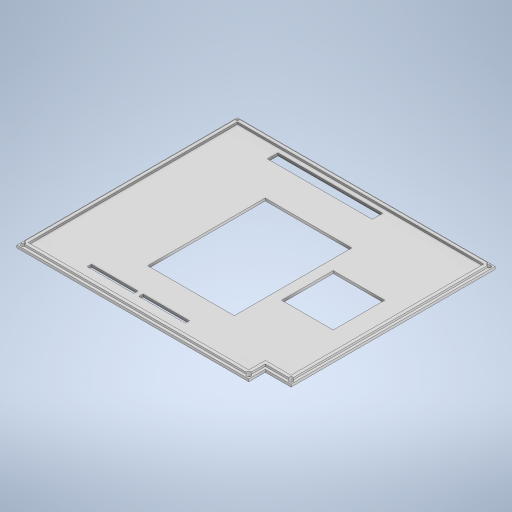
# Autodesk Inventor part: Xavier V3-1 Lid
Saved by Autodesk Inventor 2024 (Build 280153000, 153)
## iProperties
Created: 2023-11-29
Part Number: Xavier V3-1 Lid
Material: Generic
Document SubType Name: Modeling
Designer: close
Density: 1 g/cm^3
Appearance: Default
Author: close
Autodesk Inventor part; units mm, degrees
ref_plane "YZ Plane" through (0, 0, 0) normal (1, 0, 0) x (0, 1, 0)
ref_plane "XZ Plane" through (0, 0, 0) normal (0, 1, 0) x (-1, 0, 0)
ref_plane "XY Plane" through (0, 0, 0) normal (0, 0, 1) x (1, 0, 0)
sketch "Sketch1" plane through (0, 0, 0) normal (0, 1, 0) x (-1, 0, 0)
  line L0 (0, 0) -> (-112.5, 0)
  line L1 (-125, 8) -> (-125, 107)
  line L2 (-125, 107) -> (0, 107)
  line L3 (0, 107) -> (0, 0)
  line L4 (-1.5, 105.5) -> (-123.5, 105.5) construction
  line L5 (-123.5, 105.5) -> (-123.5, 9.5) construction
  line L6 (-111, 1.5) -> (-1.5, 1.5) construction
  line L7 (-1.5, 1.5) -> (-1.5, 105.5) construction
  circle A0 centre (-1.5, 1.5) radius 1
  circle A1 centre (-1.5, 105.5) radius 1
  circle A2 centre (-123.5, 105.5) radius 1
  line L8 (-109.75, 2.75) -> (-2.75, 2.75)
  line L9 (-2.75, 2.75) -> (-2.75, 104.25)
  line L10 (-2.75, 104.25) -> (-122.25, 104.25)
  line L11 (-1.25, 1.25) -> (-1.25, 105.75)
  line L12 (-1.25, 105.75) -> (-123.75, 105.75)
  line L13 (-112.5, 0) -> (-100.7656, 0)
  line L14 (-125, 16.4258) -> (-125, 8)
  line L15 (-112.5, 0) -> (-112.5, 8)
  line L16 (-112.5, 8) -> (-125, 8)
  line L17 (-111.25, 9.25) -> (-111.25, 1.25)
  line L18 (-111.25, 9.25) -> (-123.75, 9.25)
  line L19 (-123.75, 105.75) -> (-123.75, 9.25)
  line L20 (-111.25, 1.25) -> (-1.25, 1.25)
  line L21 (-109.75, 2.75) -> (-109.75, 10.75)
  line L22 (-122.25, 104.25) -> (-122.25, 10.75)
  line L23 (-109.75, 10.75) -> (-122.25, 10.75)
  line L24 (-111, 1.5) -> (-111, 9.5) construction
  line L25 (-111, 9.5) -> (-123.5, 9.5) construction
  circle A3 centre (-111, 1.5) radius 1
  circle A4 centre (-123.5, 9.5) radius 1
  point P0 (-2.4682, 105.75)
  point P1 (-1.384, 105.75)
  point P2 (-1.2818, 1.25)
  point P3 (-2.4682, 1.25)
  point P4 (-123.7182, 105.75)
  point P5 (-122.5318, 105.75)
  point P6 (-1.25, 104.5318)
  point P7 (-1.25, 2.4682)
  point P8 (-123.75, 104.5318)
  point P9 (-123.75, 10.4682)
  point P10 (-122.5318, 9.25)
  point P11 (-111.25, 2.4682)
  point P12 (-110.0318, 1.25)
  dimension "d1" = 107
  dimension "d6" = 2
  dimension "d7" = 2.75
  dimension "d9" = 2.75
  dimension "d10" = 2.75
  dimension "d13" = 1.25
  dimension "d14" = 1.25
  dimension "d29" = 125
  dimension "d31" = 8
  dimension "d33" = 2.75
  dimension "d34" = 2.75
  dimension "d35" = 1.25
  dimension "d37" = 2.75
  dimension "d38" = 1.25
  dimension "d39" = 1.25
  dimension "d40" = 12.5
  dimension "d41" = 1.25
  dimension "d42" = 1.5
  dimension "d43" = 1.5
  dimension "d44" = 1.5
  dimension "d45" = 1.5
  dimension "d46" = 1.5
  dimension "d47" = 1.5
  constraints: 52 end point, 10 parallel, 8 coincident, 7 perpendicular, 6 horizontal, 5 centre point, 4 equal radius, 1 vertical
  measures "d1" distance of L2.end L0.start
  measures "d6" diameter of A0
  measures "d7" distance between parallel lines of L0 L8
  measures "d9" distance between parallel lines of L2 L10
  measures "d10" distance between parallel lines of L3 L9
  measures "d13" distance between parallel lines of L2 L12
  measures "d14" distance between parallel lines of L3 L11
  measures "d29" distance between parallel lines of L3 L1
  measures "d31" distance of L0.end L15.end
  measures "d33" distance between parallel lines of L15 L21
  measures "d34" distance between parallel lines of L16 L23
  measures "d35" distance between parallel lines of L15 L17
  measures "d37" distance between parallel lines of L14 L22
  measures "d38" distance between parallel lines of L1 L19
  measures "d39" distance between parallel lines of L0 L20
  measures "d40" distance between parallel lines of L15 L1
  measures "d41" distance between parallel lines of L16 L18
  measures "d42" distance between parallel lines of L0 L6
  measures "d43" distance between parallel lines of L3 L7
  measures "d44" distance between parallel lines of L2 L4
  measures "d45" distance between parallel lines of L1 L5
  measures "d46" distance between parallel lines of L15 L24
  measures "d47" distance between parallel lines of L16 L25
extrude "Extrusion1" add sketch "Sketch1" along normal blind 1 contours L11 L20 A0 | A0 L20 A3 L17 L18 A4 L19 A2 L12 A1 L11 | A1 L12 L11 | L20 L17 A3 | A2 L19 L12 | L18 L19 A4 picked at (-1.8849, 1.8849) picked at (-1.8849, 105.1151) picked at (-110.6208, 1.8908) picked at (-123.1208, 105.1092) picked at (-123.1208, 9.8908)
extrude "Extrusion2" add sketch "Sketch1" against normal blind 1.25 contours L0 L15 L16 L1 L2 L3 | A0 L20 L11 | L11 L20 A0 | A0 L20 A3 L17 L18 A4 L19 A2 L12 A1 L11 | L11 L12 A1 | A1 L12 L11 | A3 L17 L20 | L20 L17 A3 | L12 L19 A2 | A2 L19 L12 | A4 L19 L18 | L18 L19 A4 | L21 L23 L22 L10 L9 L8
extrude "Extrusion3" cut sketch "Sketch1" along normal through all both and the other way through all contours A0 L20 L11 | L11 L20 A0 | L11 L12 A1 | A1 L12 L11 | A3 L17 L20 | L20 L17 A3 | L12 L19 A2 | A2 L19 L12 | A4 L19 L18 | L18 L19 A4
sketch "Sketch3" plane through (0, -1.25, 0) normal (0, -1, 0) x (1, 0, 0)
  line L0 (82.4634, 23) -> (40.4634, 23)
  line L1 (40.4634, 23) -> (40.4634, 80)
  line L2 (40.4634, 80) -> (82.4634, 80)
  line L3 (82.4634, 80) -> (82.4634, 23)
  line L4 (0, 0) -> (112.5, 0) projected
  dimension "d24" = 57
  dimension "d48" = 42
  dimension "d49" = 23
  constraints: 8 end point, 2 parallel, 1 horizontal, 1 perpendicular
  measures "d24" distance between parallel lines of L2 L0
  measures "d48" distance between parallel lines of L1 L3
  measures "d49" distance between parallel lines of L4 L0
extrude "Extrusion5" cut sketch "Sketch3" against normal up to next
ref_plane "Work Plane1" through (112.5, 0, 53.5) normal (0, 0, -1) x (-1, 0, 0)
mirror "Mirror1" about plane through (112.5, 0, 53.5) normal (0, 0, -1) remove original yes
sketch "Sketch4" plane through (0, -1.25, 0) normal (0, -1, 0) x (1, 0, 0)
  line L0 (24.6126, 4.953) -> (75.4126, 4.953)
  line L1 (75.4126, 4.953) -> (75.4126, 10.033)
  line L2 (75.4126, 10.033) -> (24.6126, 10.033)
  line L3 (24.6126, 10.033) -> (24.6126, 4.953)
  line L4 (26.2, 97) -> (48.7, 97)
  line L5 (48.7, 97) -> (48.7, 99)
  line L6 (48.7, 99) -> (26.2, 99)
  line L7 (26.2, 99) -> (26.2, 97)
  line L8 (51.2, 97) -> (73.7, 97)
  line L9 (73.7, 97) -> (73.7, 99)
  line L10 (73.7, 99) -> (51.2, 99)
  line L11 (51.2, 99) -> (51.2, 97)
  line L12 (87.4634, 41) -> (112.4634, 41)
  line L13 (112.4634, 41) -> (112.4634, 66)
  line L14 (112.4634, 66) -> (87.4634, 66)
  line L15 (87.4634, 66) -> (87.4634, 41)
  line L16 (0, 0) -> (0, 107) projected
  line L17 (0, 107) -> (112.5, 107) projected
  line L18 (125, 0) -> (0, 0) projected
  line L19 (82.4634, 27) -> (82.4634, 84) projected
  point P0 (26.2, 98)
  point P1 (73.7, 98)
  point P2 (48.7, 98)
  point P3 (51.2, 98)
  point P4 (37.45, 99)
  point P5 (37.45, 97)
  point P6 (24.6126, 7.493)
  point P7 (75.4126, 7.493)
  dimension "d50" = 26.2
  dimension "d51" = 73.7
  dimension "d52" = 2.5
  dimension "d53" = 8
  dimension "d54" = 10
  dimension "d55" = 25
  dimension "d56" = 25
  dimension "d57" = 41
  dimension "d58" = 5
  dimension "d59" = 24.6126
  dimension "d60" = 4.953
  dimension "d62" = 50.8
  dimension "d63" = 5.08
  constraints: 32 end point, 8 midpoint, 8 parallel, 4 horizontal, 4 perpendicular, 2 collinear, 1 point on line
  measures "d50" distance from line of L16 point (26.2, 98)
  measures "d51" distance from line of L16 point (73.7, 98)
  measures "d52" distance of point (48.7, 98) point (51.2, 98)
  measures "d53" distance from line of L17 point (37.45, 99)
  measures "d54" distance from line of L17 point (37.45, 97)
  measures "d55" distance of L12.end L13.end
  measures "d56" distance of L13.end L14.end
  measures "d57" distance between parallel lines of L18 L12
  measures "d58" distance between parallel lines of L19 L15
  measures "d59" distance from line of L16 point (24.613, 7.493)
  measures "d60" distance between parallel lines of L18 L0
  measures "d62" distance from line of point (75.413, 7.493) L3
  measures "d63" distance between parallel lines of L2 L0
extrude "Extrusion6" cut sketch "Sketch4" against normal through all
equation "\"d9\" = d7"
equation "\"d10\" = d9"
equation "\"d13\" = d11"
equation "\"d14\" = d11"
equation "\"d33\" = d7"
equation "\"d34\" = d33"
equation "\"d35\" = d13"
equation "\"d37\" = d34"
equation "\"d38\" = d36"
equation "\"d39\" = d36"
equation "\"d41\" = d35"
equation "\"d43\" = d42"
equation "\"d12\" = d11"
equation "\"d36\" = d35"
equation "\"d11\" = 1.25"
body "Solid1"
